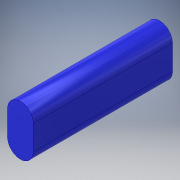
# Autodesk Inventor part: Batterie
Saved by Autodesk Inventor 2019 (Build 230136000, 136)
## iProperties
Created: 2019-07-30
Part Number: Batterie
Material: Plastique ABS
Document SubType Name: Modeling
Designer: Sébastien DI MERCURIO
Density: 1.06 g/cm^3
Appearance: Bleu - Peinture murale - Brillant
Author: Sébastien DI MERCURIO
Autodesk Inventor part; units mm, degrees
ref_plane "YZ Plane" through (0, 0, 0) normal (1, 0, 0) x (0, 1, 0)
ref_plane "XZ Plane" through (0, 0, 0) normal (0, 1, 0) x (-1, 0, 0)
ref_plane "XY Plane" through (0, 0, 0) normal (0, 0, 1) x (1, 0, 0)
sketch "Esquisse1" plane through (0, 0, 0) normal (0, 0, 1) x (1, 0, 0)
  line L0 (0, 0) -> (0, 23) construction
  line L1 (12, 0) -> (12, 23)
  line L2 (-12, 23) -> (-12, 0)
  arc A0 (-12, 0) -> (12, 0) centre (0, 0) ccw
  arc A1 (12, 23) -> (-12, 23) centre (0, 23) ccw
  point P0 (0, 11.5)
  dimension "d0" = 47
  dimension "d1" = 24
  constraints: 8 end point, 4 point on circle, 4 tangent, 2 centre point, 1 midpoint, 1 parallel, 1 vertical
  measures "d1" distance between parallel lines of L1 L2
extrude "Extrusion1" add sketch "Esquisse1" along normal blind 130
